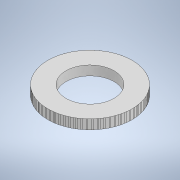
# Autodesk Inventor part: just_ring
Saved by Autodesk Inventor 2021 (Build 250183000, 183)
## iProperties
Created: 2021-03-25
Part Number: just_ring
Material: Generic
Document SubType Name: Modeling
Designer: Patrick
Density: 1 g/cm^3
Appearance: Default
Author: Patrick
Autodesk Inventor part; units mm, degrees
ref_plane "YZ Plane" through (0, 0, 0) normal (1, 0, 0) x (0, 1, 0)
ref_plane "XZ Plane" through (0, 0, 0) normal (0, 1, 0) x (-1, 0, 0)
ref_plane "XY Plane" through (0, 0, 0) normal (0, 0, 1) x (1, 0, 0)
sketch "Sketch1" plane through (0, 0, 0) normal (0, 1, 0) x (-1, 0, 0)
  line L0 (-12.629, -4.2945) -> (-13.1433, -4.6896)
  line L1 (-13.1433, -4.6896) -> (-14.2641, -5.6054)
  line L2 (-14.2641, -5.6054) -> (-14.7541, -6.0486)
  line L3 (-14.7541, -6.0486) -> (-15.7734, -7.0678)
  line L4 (-15.7734, -7.0678) -> (-16.2233, -7.5456)
  line L5 (-16.2233, -7.5456) -> (-17.0958, -8.6087)
  line L6 (-17.0958, -8.6087) -> (-17.4933, -9.1029)
  line L7 (-17.4933, -9.1029) -> (-17.8535, -9.6283)
  line L8 (-17.8535, -9.6283) -> (-18.6167, -10.7652)
  line L9 (-18.6167, -10.7652) -> (-18.9508, -11.3448)
  line L10 (-18.9508, -11.3448) -> (-19.6231, -12.5962)
  line L11 (-19.6231, -12.5962) -> (-19.916, -13.2137)
  line L12 (-19.916, -13.2137) -> (-20.4563, -14.518)
  line L13 (-20.4563, -14.518) -> (-20.6978, -15.1543)
  line L14 (-20.6978, -15.1543) -> (-21.0881, -16.4409)
  line L15 (-21.0881, -16.4409) -> (-21.2732, -17.0733)
  line L16 (-21.2732, -17.0733) -> (-21.4103, -17.7219)
  line L17 (-21.4103, -17.7219) -> (-21.6738, -19.0321)
  line L18 (-21.6738, -19.0321) -> (-21.7643, -19.7234)
  line L19 (-21.7643, -19.7234) -> (-21.903, -21.1009)
  line L20 (-21.903, -21.1009) -> (-21.9387, -21.8132)
  line L21 (-21.9387, -21.8132) -> (-21.9389, -23.1874)
  line L22 (-21.9389, -23.1874) -> (-21.9175, -23.8979)
  line L23 (-21.9175, -23.8979) -> (-21.7894, -25.199)
  line L24 (-21.7894, -25.199) -> (-21.7152, -25.8835)
  line L25 (-21.7152, -25.8835) -> (-21.5881, -26.5648)
  line L26 (-21.5881, -26.5648) -> (-21.3375, -27.8389)
  line L27 (-21.3375, -27.8389) -> (-21.1484, -28.5428)
  line L28 (-21.1484, -28.5428) -> (-20.7609, -29.8303)
  line L29 (-20.7609, -29.8303) -> (-20.5105, -30.5323)
  line L30 (-20.5105, -30.5323) -> (-19.9999, -31.7651)
  line L31 (-19.9999, -31.7651) -> (-19.6954, -32.4421)
  line L32 (-19.6954, -32.4421) -> (-19.0969, -33.5619)
  line L33 (-19.0969, -33.5619) -> (-18.752, -34.1922)
  line L34 (-18.752, -34.1922) -> (-18.3577, -34.7979)
  line L35 (-18.3577, -34.7979) -> (-17.6592, -35.8481)
  line L36 (-17.6592, -35.8481) -> (-17.1966, -36.4501)
  line L37 (-17.1966, -36.4501) -> (-16.3697, -37.4621)
  line L38 (-16.3697, -37.4621) -> (-15.8498, -38.0369)
  line L39 (-15.8498, -38.0369) -> (-14.9319, -38.955)
  line L40 (-14.9319, -38.955) -> (-14.3709, -39.4832)
  line L41 (-14.3709, -39.4832) -> (-13.4148, -40.268)
  line L42 (-13.4148, -40.268) -> (-12.8349, -40.7344)
  line L43 (-12.8349, -40.7344) -> (-12.2182, -41.1571)
  line L44 (-12.2182, -41.1571) -> (-11.1966, -41.8429)
  line L45 (-11.1966, -41.8429) -> (-10.5179, -42.2342)
  line L46 (-10.5179, -42.2342) -> (-9.3928, -42.8387)
  line L47 (-9.3928, -42.8387) -> (-8.672, -43.1805)
  line L48 (-8.672, -43.1805) -> (-7.4973, -43.6671)
  line L49 (-7.4973, -43.6671) -> (-6.7577, -43.9478)
  line L50 (-6.7577, -43.9478) -> (-5.5958, -44.3003)
  line L51 (-5.5958, -44.3003) -> (-4.8646, -44.5142)
  line L52 (-4.8646, -44.5142) -> (-4.1173, -44.6722)
  line L53 (-4.1173, -44.6722) -> (-2.9304, -44.9109)
  line L54 (-2.9304, -44.9109) -> (-2.1392, -45.0145)
  line L55 (-2.1392, -45.0145) -> (-0.8854, -45.1407)
  line L56 (-0.8854, -45.1407) -> (-0.0764, -45.1813)
  line L57 (-0.0764, -45.1813) -> (1.1817, -45.1813)
  line L58 (1.1817, -45.1813) -> (1.982, -45.1573)
  line L59 (1.982, -45.1573) -> (3.1812, -45.0392)
  line L60 (3.1812, -45.0392) -> (3.9454, -44.9563)
  line L61 (3.9454, -44.9563) -> (4.7012, -44.8153)
  line L62 (4.7012, -44.8153) -> (5.8835, -44.5827)
  line L63 (5.8835, -44.5827) -> (6.6567, -44.375)
  line L64 (6.6567, -44.375) -> (7.8614, -44.0123)
  line L65 (7.8614, -44.0123) -> (8.6244, -43.7402)
  line L66 (8.6244, -43.7402) -> (9.7886, -43.258)
  line L67 (9.7886, -43.258) -> (10.5163, -42.9307)
  line L68 (10.5163, -42.9307) -> (11.584, -42.36)
  line L69 (11.584, -42.36) -> (12.254, -41.9933)
  line L70 (12.254, -41.9933) -> (12.8925, -41.5776)
  line L71 (12.8925, -41.5776) -> (13.9035, -40.9052)
  line L72 (13.9035, -40.9052) -> (14.5308, -40.4232)
  line L73 (14.5308, -40.4232) -> (15.5153, -39.6186)
  line L74 (15.5153, -39.6186) -> (16.107, -39.0835)
  line L75 (16.107, -39.0835) -> (17.0101, -38.1804)
  line L76 (17.0101, -38.1804) -> (17.5472, -37.61)
  line L77 (17.5472, -37.61) -> (18.3278, -36.6589)
  line L78 (18.3278, -36.6589) -> (18.7964, -36.0763)
  line L79 (18.7964, -36.0763) -> (19.2172, -35.4625)
  line L80 (19.2172, -35.4625) -> (19.9065, -34.4355)
  line L81 (19.9065, -34.4355) -> (20.2914, -33.7679)
  line L82 (20.2914, -33.7679) -> (20.9057, -32.6242)
  line L83 (20.9057, -32.6242) -> (21.2378, -31.924)
  line L84 (21.2378, -31.924) -> (21.7379, -30.7165)
  line L85 (21.7379, -30.7165) -> (22.0073, -30.0068)
  line L86 (22.0073, -30.0068) -> (22.3734, -28.7998)
  line L87 (22.3734, -28.7998) -> (22.5764, -28.1061)
  line L88 (22.5764, -28.1061) -> (22.725, -27.4032)
  line L89 (22.725, -27.4032) -> (22.9752, -26.1584)
  line L90 (22.9752, -26.1584) -> (23.0717, -25.4223)
  line L91 (23.0717, -25.4223) -> (23.2052, -24.0947)
  line L92 (23.2052, -24.0947) -> (23.2425, -23.3503)
  line L93 (23.2425, -23.3503) -> (23.2425, -22.0057)
  line L94 (23.2425, -22.0057) -> (23.2206, -21.2772)
  line L95 (23.2206, -21.2772) -> (23.0933, -19.9849)
  line L96 (23.0933, -19.9849) -> (23.0186, -19.296)
  line L97 (23.0186, -19.296) -> (22.8924, -18.6191)
  line L98 (22.8924, -18.6191) -> (22.6399, -17.3363)
  line L99 (22.6399, -17.3363) -> (22.4555, -16.6498)
  line L100 (22.4555, -16.6498) -> (22.0593, -15.334)
  line L101 (22.0593, -15.334) -> (21.8198, -14.6623)
  line L102 (21.8198, -14.6623) -> (21.2899, -13.3832)
  line L103 (21.2899, -13.3832) -> (21.0039, -12.7473)
  line L104 (21.0039, -12.7473) -> (20.3739, -11.5687)
  line L105 (20.3739, -11.5687) -> (20.0557, -10.9872)
  line L106 (20.0557, -10.9872) -> (19.6961, -10.435)
  line L107 (19.6961, -10.435) -> (18.9515, -9.3155)
  line L108 (18.9515, -9.3155) -> (18.5368, -8.7758)
  line L109 (18.5368, -8.7758) -> (17.6434, -7.6826)
  line L110 (17.6434, -7.6826) -> (17.185, -7.1757)
  line L111 (17.185, -7.1757) -> (16.1805, -6.1713)
  line L112 (16.1805, -6.1713) -> (15.6934, -5.7126)
  line L113 (15.6934, -5.7126) -> (14.635, -4.844)
  line L114 (14.635, -4.844) -> (14.1386, -4.4447)
  line L115 (14.1386, -4.4447) -> (13.6155, -4.0861)
  line L116 (13.6155, -4.0861) -> (12.4736, -3.3197)
  line L117 (12.4736, -3.3197) -> (11.905, -2.9919)
  line L118 (11.905, -2.9919) -> (10.6351, -2.3098)
  line L119 (10.6351, -2.3098) -> (10.0382, -2.0266)
  line L120 (10.0382, -2.0266) -> (8.701, -1.4728)
  line L121 (8.701, -1.4728) -> (8.0947, -1.2427)
  line L122 (8.0947, -1.2427) -> (6.7627, -0.8386)
  line L123 (6.7627, -0.8386) -> (6.1803, -0.6682)
  arc A0 (6.1803, -0.6682) -> (6.1557, -0.662) centre (0.6527, -22.5966) ccw
  line L124 (6.1557, -0.662) -> (5.5636, -0.5369)
  line L125 (5.5636, -0.5369) -> (4.1958, -0.2619)
  line L126 (4.1958, -0.2619) -> (3.5595, -0.1785)
  line L127 (3.5595, -0.1785) -> (2.1083, -0.0325)
  line L128 (2.1083, -0.0325) -> (1.4607, 0)
  line L129 (1.4607, 0) -> (0, 0)
  line L130 (0, 0) -> (-0.6387, -0.0192)
  line L131 (-0.6387, -0.0192) -> (-2.0329, -0.1565)
  line L132 (-2.0329, -0.1565) -> (-2.6148, -0.2196)
  arc A1 (-2.6148, -0.2196) -> (-2.6691, -0.2276) centre (0.6527, -22.5966) ccw
  line L133 (-2.6691, -0.2276) -> (-3.2445, -0.3349)
  line L134 (-3.2445, -0.3349) -> (-4.6191, -0.6053)
  line L135 (-4.6191, -0.6053) -> (-5.2362, -0.7711)
  line L136 (-5.2362, -0.7711) -> (-6.6349, -1.1922)
  line L137 (-6.6349, -1.1922) -> (-7.2456, -1.41)
  line L138 (-7.2456, -1.41) -> (-8.5932, -1.9681)
  line L139 (-8.5932, -1.9681) -> (-9.1784, -2.2314)
  line L140 (-9.1784, -2.2314) -> (-10.4089, -2.889)
  line L141 (-10.4089, -2.889) -> (-10.9398, -3.1795)
  arc A2 (-10.9398, -3.1795) -> (-10.9616, -3.1926) centre (0.6527, -22.5966) ccw
  line L142 (-10.9616, -3.1926) -> (-11.4701, -3.5236)
  line L143 (-11.4701, -3.5236) -> (-12.629, -4.2945)
  circle A3 centre (0.6527, -22.5966) radius 12.9
  circle A4 centre (-8.75, -38.068) radius 4.3815
  circle A5 centre (-15.226, -31.2939) radius 4.3815
  circle A6 centre (-17.4473, -22.1894) radius 4.3815
  circle A7 centre (-14.8187, -13.1939) radius 4.3815
  circle A8 centre (0.2455, -40.6966) radius 4.3815
  circle A9 centre (9.35, -38.4753) radius 4.3815
  circle A10 centre (16.1242, -31.9993) radius 4.3815
  circle A11 centre (1.0599, -4.4966) radius 4.3815
  circle A12 centre (-8.0446, -6.7179) radius 4.3815
  circle A13 centre (10.0554, -7.1251) radius 4.3815
  circle A14 centre (18.7527, -23.0038) radius 4.3815
  circle A15 centre (16.5314, -13.8993) radius 4.3815
  point P0 (0, 0)
  point P1 (0.6527, -22.5966)
  constraints: 288 end point, 16 centre point, 6 point on circle
extrude "Extrusion1" add sketch "Sketch1" along normal blind 2.54
sketch "Sketch2" plane through (0, 2.54, 0) normal (0, 1, 0) x (1, 0, 0)
  line L0 (21.6738, 19.0321) -> (21.7643, 19.7234) projected
  line L1 (21.7643, 19.7234) -> (21.903, 21.1009) projected
  line L2 (21.903, 21.1009) -> (21.9387, 21.8132) projected
  line L3 (21.9387, 21.8132) -> (21.9389, 23.1874) projected
  line L4 (21.9389, 23.1874) -> (21.9175, 23.8979) projected
  line L5 (21.9175, 23.8979) -> (21.7894, 25.199) projected
  line L6 (21.7894, 25.199) -> (21.7152, 25.8835) projected
  line L7 (21.7152, 25.8835) -> (21.5881, 26.5648) projected
  line L8 (21.5881, 26.5648) -> (21.3375, 27.8389) projected
  line L9 (21.3375, 27.8389) -> (21.1484, 28.5428) projected
  line L10 (21.1484, 28.5428) -> (20.7609, 29.8303) projected
  line L11 (20.7609, 29.8303) -> (20.5105, 30.5323) projected
  line L12 (20.5105, 30.5323) -> (19.9999, 31.7651) projected
  line L13 (19.9999, 31.7651) -> (19.6954, 32.4421) projected
  line L14 (19.6954, 32.4421) -> (19.0969, 33.5619) projected
  line L15 (19.0969, 33.5619) -> (18.752, 34.1922) projected
  line L16 (18.752, 34.1922) -> (18.3577, 34.7979) projected
  line L17 (18.3577, 34.7979) -> (17.6592, 35.8481) projected
  line L18 (17.6592, 35.8481) -> (17.1966, 36.4501) projected
  line L19 (17.1966, 36.4501) -> (16.3697, 37.4621) projected
  line L20 (16.3697, 37.4621) -> (15.8498, 38.0369) projected
  line L21 (15.8498, 38.0369) -> (14.9319, 38.955) projected
  line L22 (14.9319, 38.955) -> (14.3709, 39.4832) projected
  line L23 (14.3709, 39.4832) -> (13.4148, 40.268) projected
  line L24 (13.4148, 40.268) -> (12.8349, 40.7344) projected
  line L25 (12.8349, 40.7344) -> (12.2182, 41.1571) projected
  line L26 (12.2182, 41.1571) -> (11.1966, 41.8429) projected
  line L27 (11.1966, 41.8429) -> (10.5179, 42.2342) projected
  line L28 (10.5179, 42.2342) -> (9.3928, 42.8387) projected
  line L29 (9.3928, 42.8387) -> (8.672, 43.1805) projected
  line L30 (8.672, 43.1805) -> (7.4973, 43.6671) projected
  line L31 (7.4973, 43.6671) -> (6.7577, 43.9478) projected
  line L32 (6.7577, 43.9478) -> (5.5958, 44.3003) projected
  line L33 (5.5958, 44.3003) -> (4.8646, 44.5142) projected
  line L34 (4.8646, 44.5142) -> (4.1173, 44.6722) projected
  line L35 (4.1173, 44.6722) -> (2.9304, 44.9109) projected
  line L36 (2.9304, 44.9109) -> (2.1392, 45.0145) projected
  line L37 (2.1392, 45.0145) -> (0.8854, 45.1407) projected
  line L38 (0.8854, 45.1407) -> (0.0764, 45.1813) projected
  line L39 (0.0764, 45.1813) -> (-1.1817, 45.1813) projected
  line L40 (-1.1817, 45.1813) -> (-1.982, 45.1573) projected
  line L41 (-1.982, 45.1573) -> (-3.1812, 45.0392) projected
  line L42 (-3.1812, 45.0392) -> (-3.9454, 44.9563) projected
  line L43 (-3.9454, 44.9563) -> (-4.7012, 44.8153) projected
  line L44 (-4.7012, 44.8153) -> (-5.8835, 44.5827) projected
  line L45 (-5.8835, 44.5827) -> (-6.6567, 44.375) projected
  line L46 (-6.6567, 44.375) -> (-7.8614, 44.0123) projected
  line L47 (-7.8614, 44.0123) -> (-8.6244, 43.7402) projected
  line L48 (-8.6244, 43.7402) -> (-9.7886, 43.258) projected
  line L49 (-9.7886, 43.258) -> (-10.5163, 42.9307) projected
  line L50 (-10.5163, 42.9307) -> (-11.584, 42.36) projected
  line L51 (-11.584, 42.36) -> (-12.254, 41.9933) projected
  line L52 (-12.254, 41.9933) -> (-12.8925, 41.5776) projected
  line L53 (-12.8925, 41.5776) -> (-13.9035, 40.9052) projected
  line L54 (-13.9035, 40.9052) -> (-14.5308, 40.4232) projected
  line L55 (-14.5308, 40.4232) -> (-15.5153, 39.6186) projected
  line L56 (-15.5153, 39.6186) -> (-16.107, 39.0835) projected
  line L57 (-16.107, 39.0835) -> (-17.0101, 38.1804) projected
  line L58 (-17.0101, 38.1804) -> (-17.5472, 37.61) projected
  line L59 (-17.5472, 37.61) -> (-18.3278, 36.6589) projected
  line L60 (-18.3278, 36.6589) -> (-18.7964, 36.0763) projected
  line L61 (-18.7964, 36.0763) -> (-19.2172, 35.4625) projected
  line L62 (-19.2172, 35.4625) -> (-19.9065, 34.4355) projected
  line L63 (-19.9065, 34.4355) -> (-20.2914, 33.7679) projected
  line L64 (-20.2914, 33.7679) -> (-20.9057, 32.6242) projected
  line L65 (-20.9057, 32.6242) -> (-21.2378, 31.924) projected
  line L66 (-21.2378, 31.924) -> (-21.7379, 30.7165) projected
  line L67 (-21.7379, 30.7165) -> (-22.0073, 30.0068) projected
  line L68 (-22.0073, 30.0068) -> (-22.3734, 28.7998) projected
  line L69 (-22.3734, 28.7998) -> (-22.5764, 28.1061) projected
  line L70 (-22.5764, 28.1061) -> (-22.725, 27.4032) projected
  line L71 (-22.725, 27.4032) -> (-22.9752, 26.1584) projected
  line L72 (-22.9752, 26.1584) -> (-23.0717, 25.4223) projected
  line L73 (-23.0717, 25.4223) -> (-23.2052, 24.0947) projected
  line L74 (-23.2052, 24.0947) -> (-23.2425, 23.3503) projected
  line L75 (-23.2425, 23.3503) -> (-23.2425, 22.0057) projected
  line L76 (-23.2425, 22.0057) -> (-23.2206, 21.2772) projected
  line L77 (-23.2206, 21.2772) -> (-23.0933, 19.9849) projected
  line L78 (-23.0933, 19.9849) -> (-23.0186, 19.296) projected
  line L79 (-23.0186, 19.296) -> (-22.8924, 18.6191) projected
  line L80 (-22.8924, 18.6191) -> (-22.6399, 17.3363) projected
  line L81 (-22.6399, 17.3363) -> (-22.4555, 16.6498) projected
  line L82 (-22.4555, 16.6498) -> (-22.0593, 15.334) projected
  line L83 (-22.0593, 15.334) -> (-21.8198, 14.6623) projected
  line L84 (-21.8198, 14.6623) -> (-21.2899, 13.3832) projected
  line L85 (-21.2899, 13.3832) -> (-21.0039, 12.7473) projected
  line L86 (-21.0039, 12.7473) -> (-20.3739, 11.5687) projected
  line L87 (-20.3739, 11.5687) -> (-20.0557, 10.9872) projected
  line L88 (-20.0557, 10.9872) -> (-19.6961, 10.435) projected
  line L89 (-19.6961, 10.435) -> (-18.9515, 9.3155) projected
  line L90 (-18.9515, 9.3155) -> (-18.5368, 8.7758) projected
  line L91 (-18.5368, 8.7758) -> (-17.6434, 7.6826) projected
  line L92 (-17.6434, 7.6826) -> (-17.185, 7.1757) projected
  line L93 (-17.185, 7.1757) -> (-16.1805, 6.1713) projected
  line L94 (-16.1805, 6.1713) -> (-15.6934, 5.7126) projected
  line L95 (-15.6934, 5.7126) -> (-14.635, 4.844) projected
  line L96 (-14.635, 4.844) -> (-14.1386, 4.4447) projected
  line L97 (-14.1386, 4.4447) -> (-13.6155, 4.0861) projected
  line L98 (-13.6155, 4.0861) -> (-12.4736, 3.3197) projected
  line L99 (-12.4736, 3.3197) -> (-11.905, 2.9919) projected
  line L100 (-11.905, 2.9919) -> (-10.6351, 2.3098) projected
  line L101 (-10.6351, 2.3098) -> (-10.0382, 2.0266) projected
  line L102 (-10.0382, 2.0266) -> (-8.701, 1.4728) projected
  line L103 (-8.701, 1.4728) -> (-8.0947, 1.2427) projected
  line L104 (-8.0947, 1.2427) -> (-6.7627, 0.8386) projected
  line L105 (-6.7627, 0.8386) -> (-6.1803, 0.6682) projected
  arc A0 (-6.1803, 0.6682) -> (-6.1557, 0.662) centre (-0.6527, 22.5966) ccw projected
  line L106 (-6.1557, 0.662) -> (-5.5636, 0.5369) projected
  line L107 (-5.5636, 0.5369) -> (-4.1958, 0.2619) projected
  line L108 (-4.1958, 0.2619) -> (-3.5595, 0.1785) projected
  line L109 (-3.5595, 0.1785) -> (-2.1083, 0.0325) projected
  line L110 (-2.1083, 0.0325) -> (-1.4607, 0) projected
  line L111 (-1.4607, 0) -> (0, 0) projected
  line L112 (0, 0) -> (0.6387, 0.0192) projected
  line L113 (0.6387, 0.0192) -> (2.0329, 0.1565) projected
  line L114 (2.0329, 0.1565) -> (2.6148, 0.2196) projected
  arc A1 (2.6148, 0.2196) -> (2.6691, 0.2276) centre (-0.6527, 22.5966) ccw projected
  line L115 (2.6691, 0.2276) -> (3.2445, 0.3349) projected
  line L116 (3.2445, 0.3349) -> (4.6191, 0.6053) projected
  line L117 (4.6191, 0.6053) -> (5.2362, 0.7711) projected
  line L118 (5.2362, 0.7711) -> (6.6349, 1.1922) projected
  line L119 (6.6349, 1.1922) -> (7.2456, 1.41) projected
  line L120 (7.2456, 1.41) -> (8.5932, 1.9681) projected
  line L121 (8.5932, 1.9681) -> (9.1784, 2.2314) projected
  line L122 (9.1784, 2.2314) -> (10.4089, 2.889) projected
  line L123 (10.4089, 2.889) -> (10.9398, 3.1795) projected
  arc A2 (10.9398, 3.1795) -> (10.9616, 3.1926) centre (-0.6527, 22.5966) ccw projected
  line L124 (10.9616, 3.1926) -> (11.4701, 3.5236) projected
  line L125 (11.4701, 3.5236) -> (12.629, 4.2945) projected
  line L126 (12.629, 4.2945) -> (13.1433, 4.6896) projected
  line L127 (13.1433, 4.6896) -> (14.2641, 5.6054) projected
  line L128 (14.2641, 5.6054) -> (14.7541, 6.0486) projected
  line L129 (14.7541, 6.0486) -> (15.7734, 7.0678) projected
  line L130 (15.7734, 7.0678) -> (16.2233, 7.5456) projected
  line L131 (16.2233, 7.5456) -> (17.0958, 8.6087) projected
  line L132 (17.0958, 8.6087) -> (17.4933, 9.1029) projected
  line L133 (17.4933, 9.1029) -> (17.8535, 9.6283) projected
  line L134 (17.8535, 9.6283) -> (18.6167, 10.7652) projected
  line L135 (18.6167, 10.7652) -> (18.9508, 11.3448) projected
  line L136 (18.9508, 11.3448) -> (19.6231, 12.5962) projected
  line L137 (19.6231, 12.5962) -> (19.916, 13.2137) projected
  line L138 (19.916, 13.2137) -> (20.4563, 14.518) projected
  line L139 (20.4563, 14.518) -> (20.6978, 15.1543) projected
  line L140 (20.6978, 15.1543) -> (21.0881, 16.4409) projected
  line L141 (21.0881, 16.4409) -> (21.2732, 17.0733) projected
  line L142 (21.2732, 17.0733) -> (21.4103, 17.7219) projected
  line L143 (21.4103, 17.7219) -> (21.6738, 19.0321) projected
  circle A3 centre (8.75, 38.068) radius 4.3815 projected
  circle A4 centre (-1.0599, 4.4966) radius 4.3815 projected
  circle A5 centre (-10.0554, 7.1251) radius 4.3815 projected
  circle A6 centre (-16.1242, 31.9993) radius 4.3815 projected
  circle A7 centre (15.226, 31.2939) radius 4.3815 projected
  circle A8 centre (14.8187, 13.1939) radius 4.3815 projected
  circle A9 centre (8.0446, 6.7179) radius 4.3815 projected
  circle A10 centre (-18.7527, 23.0038) radius 4.3815 projected
  circle A11 centre (-16.5314, 13.8993) radius 4.3815 projected
  circle A12 centre (-9.35, 38.4753) radius 4.3815 projected
  circle A13 centre (-0.2455, 40.6966) radius 4.3815 projected
  circle A14 centre (17.4473, 22.1894) radius 4.3815 projected
  circle A15 centre (-0.6527, 22.5966) radius 12.9 projected
extrude "Extrusion2" add sketch "Sketch2" along normal blind 2.54 contours L143 L142 L141 L140 L139 L138 L137 L136 L135 L134 L133 L132 L131 L130 L129 L128 L127 L126 L125 L124 A2 L123 L122 L121 L120 L119 L118 L117 L116 L115 A1 L114 L113 L112 L111 L110 L109 L108 L107 L106 A0 L105 L104 L103 L102 L101 L100 L99 L98 L97 L96 L95 L94 L93 L92 L91 L90 L89 L88 L87 L86 L85 L84 L83 L82 L81 L80 L79 L78 L77 L76 L75 L74 L73 L72 L71 L70 L69 L68 L67 L66 L65 L64 L63 L62 L61 L60 L59 L58 L57 L56 L55 L54 L53 L52 L51 L50 L49 L48 L47 L46 L45 L44 L43 L42 L41 L40 L39 L38 L37 L36 L35 L34 L33 L32 L31 L30 L29 L28 L27 L26 L25 L24 L23 L22 L21 L20 L19 L18 L17 L16 L15 L14 L13 L12 L11 L10 L9 L8 L7 L6 L5 L4 L3 L2 L1 L0 | A3 | A4 | A5 | A6 | A7 | A8 | A9 | A10 | A11 | A12 | A13 | A14
body "Solid1"
